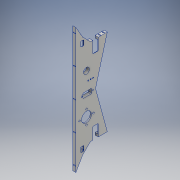
# Autodesk Inventor part: 옆판_오른쪽
Saved by Autodesk Inventor 2017 (Build 210142000, 142)
## iProperties
Part Number: 옆판_오른쪽
Material: 알루미늄 6061
Document SubType Name: Modeling
Designer: minom
Density: 2.7 g/cm^3
Appearance: 알루미늄 - 평지
Mass: 106.182 g
Surface Area: 461.014 cm^2
Volume: 39.3265 cm^3
Author: minom
Autodesk Inventor part; units mm, degrees
(part 1 of 2)
ref_plane "YZ Plane" through (0, 0, 0) normal (1, 0, 0) x (0, 1, 0)
ref_plane "XZ Plane" through (0, 0, 0) normal (0, 1, 0) x (-1, 0, 0)
ref_plane "XY Plane" through (0, 0, 0) normal (0, 0, 1) x (1, 0, 0)
sketch "스케치1" plane through (0, 0, 0) normal (1, 0, 0) x (0, 1, 0)
  line L0 (0, 0) -> (0, -320)
  line L1 (0, 0) -> (0, -50)
  line L2 (0, -50) -> (80, -50)
  line L3 (0, -320) -> (0, -270)
  line L4 (0, -270) -> (80, -270)
  line L5 (0, 0) -> (0, -30)
  line L6 (0, -30) -> (0, -50)
  line L7 (0, -320) -> (0, -290)
  line L8 (0, -290) -> (0, -270)
  line L9 (0, -290) -> (60, -290)
  line L10 (0, 0) -> (17.3205, -30)
  line L11 (0, 0) -> (34.641, 0) construction
  line L12 (17.3205, -30) -> (37.3205, -50)
  line L13 (17.3205, -30) -> (45.6048, -30) construction
  line L14 (0, -320) -> (17.3205, -290)
  line L15 (0, -320) -> (34.641, -320) construction
  line L16 (17.3205, -290) -> (37.3205, -270)
  line L17 (17.3205, -290) -> (45.6048, -290) construction
  line L18 (0, -30) -> (60, -30)
  line L19 (80, -270) -> (80, -50)
  line L20 (50, -50) -> (50, -270)
  line L21 (50, -160) -> (0, -160)
  dimension "d0" = 320
  dimension "d1" = 50
  dimension "d2" = 80
  dimension "d3" = 50
  dimension "d4" = 80
  dimension "d5" = 30
  dimension "d6" = 30
  dimension "d7" = 60
  dimension "d8" = 60
  dimension "d9" = 45
  dimension "d10" = 60
  dimension "d11" = 45
  dimension "d182" = 50
  constraints: 44 end point, 9 point on line, 6 horizontal, 4 equal length, 3 perpendicular, 2 collinear, 2 midpoint, 1 vertical
  measures "d0" distance of L0.start L0.end
  measures "d1" distance of L0.start L1.end
  measures "d2" distance of L1.end L2.end
  measures "d3" distance of L0.end L3.end
  measures "d4" distance of L3.end L4.end
  measures "d5" distance of L0.start L5.end
  measures "d6" distance of L0.end L7.end
  measures "d7" distance of L7.end L9.end
  measures "d8" angle of L10 L11
  measures "d9" angle of L12 L13
  measures "d10" angle of L15 L14
  measures "d11" angle of L17 L16
  measures "d182" distance between parallel lines of L20 L0
extrude "돌출1" add sketch "스케치1" along normal blind 8
sketch "스케치5" plane through (0, 0, 0) normal (-1, 0, 0) x (0, 0, 1)
  line L0 (-270, 80) -> (-50, 80) projected
  line L1 (-270, 80) -> (-211, 80)
  line L2 (-211, 80) -> (-211, 27)
  circle A0 centre (-211, 27) radius 21.25
  line L3 (0, 0) -> (-320, 0) projected
  dimension "d39" = 59
  dimension "d41" = 42.5
  dimension "d184" = 27
  constraints: 4 end point, 1 centre point, 1 coincident, 1 perpendicular, 1 point on line
  measures "d39" distance of L0.start L1.end
  measures "d41" diameter of A0
  measures "d184" distance from line of L3 L2.end
extrude "돌출4" cut sketch "스케치5" against normal blind 5
sketch "스케치6" plane through (5, 27, -211) normal (-1, 0, 0) x (0, 0, 1)
  circle A0 centre (0, 0) radius 21.25 projected
  line L0 (-109, -27) -> (-79, -9.6795) projected
  line L1 (211, -27) -> (-109, -27) projected
  line L2 (181, -9.6795) -> (211, -27) projected
  line L3 (161, 10.3205) -> (181, -9.6795) projected
  line L4 (161, 53) -> (161, 10.3205) projected
  line L5 (-59, 53) -> (161, 53) projected
  line L6 (-59, 10.3205) -> (-59, 53) projected
  line L7 (-79, -9.6795) -> (-59, 10.3205) projected
  line L8 (0, 0) -> (0, 17.6)
  line L9 (0, 17.6) -> (0, -17.6)
  line L10 (0, 0) -> (17.6, 0)
  line L11 (17.6, 0) -> (-17.6, 0)
  circle A1 centre (0, 17.6) radius 2.1
  circle A2 centre (17.6, 0) radius 2.1
  circle A3 centre (0, -17.6) radius 2.1
  circle A4 centre (-17.6, 0) radius 2.1
  circle A5 centre (0, 0) radius 12.6
  dimension "d44" = 17.6
  dimension "d45" = 35.2
  dimension "d46" = 17.6
  dimension "d47" = 35.2
  dimension "d48" = 4.2
  dimension "d49" = 4.2
  dimension "d50" = 4.2
  dimension "d51" = 4.2
  dimension "d52" = 25.2
  constraints: 8 end point, 5 centre point, 5 coincident, 2 point on line, 1 horizontal, 1 vertical
  measures "d44" distance of L8.start L8.end
  measures "d45" distance of L8.end L9.end
  measures "d46" distance of L8.start L10.end
  measures "d47" distance of L10.end L11.end
  measures "d48" diameter of A1
  measures "d49" diameter of A2
  measures "d50" diameter of A3
  measures "d51" diameter of A4
  measures "d52" diameter of A5
extrude "돌출5" cut sketch "스케치6" against normal blind 3 contours L11 A5 L8 | L10 A5 L9 | L8 A5 L10 | L9 A5 L11 | A1 | A2 | A3 | A4
sketch "스케치7" plane through (8, 0, 0) normal (1, 0, 0) x (0, 0, -1)
  line L0 (320, 0) -> (290, 17.3205) projected
  line L1 (290, 17.3205) -> (270, 37.3205) projected
  line L2 (270, 37.3205) -> (270, 80) projected
  line L3 (270, 80) -> (50, 80) projected
  line L4 (50, 80) -> (50, 37.3205) projected
  line L5 (50, 37.3205) -> (30, 17.3205) projected
  line L6 (30, 17.3205) -> (0, 0) projected
  line L7 (0, 0) -> (320, 0) projected
  line L8 (270, 37.3205) -> (270, 20.3205)
  line L9 (272, 20.3205) -> (281, 20.3205)
  line L10 (283, 18.3205) -> (283, 14.3205)
  line L11 (281, 12.3205) -> (272, 12.3205)
  line L12 (270, 14.3205) -> (270, 18.3205)
  line L13 (50, 37.3205) -> (50, 20.3205)
  line L14 (48, 20.3205) -> (39, 20.3205)
  line L15 (37, 18.3205) -> (37, 14.3205)
  line L16 (39, 12.3205) -> (48, 12.3205)
  line L17 (50, 14.3205) -> (50, 18.3205)
  arc A0 (39, 20.3205) -> (37, 18.3205) centre (39, 18.3205) ccw
  arc A1 (50, 18.3205) -> (48, 20.3205) centre (48, 18.3205) ccw
  arc A2 (48, 12.3205) -> (50, 14.3205) centre (48, 14.3205) ccw
  arc A3 (37, 14.3205) -> (39, 12.3205) centre (39, 14.3205) ccw
  arc A4 (272, 20.3205) -> (270, 18.3205) centre (272, 18.3205) ccw
  arc A5 (283, 18.3205) -> (281, 20.3205) centre (281, 18.3205) ccw
  arc A6 (281, 12.3205) -> (283, 14.3205) centre (281, 14.3205) ccw
  arc A7 (270, 14.3205) -> (272, 12.3205) centre (272, 14.3205) ccw
  point P0 (50, 12.3205)
  point P1 (37, 12.3205)
  point P2 (37, 20.3205)
  point P3 (270, 37.3205)
  point P4 (270, 12.3205)
  point P5 (283, 12.3205)
  point P6 (283, 20.3205)
  dimension "d55" = 17
  dimension "d56" = 8
  dimension "d57" = 13
  dimension "d61" = 17
  dimension "d62" = 13
  dimension "d63" = 8
  dimension "d142" = 2
  constraints: 20 end point, 18 point on line, 16 point on circle, 16 tangent, 8 centre point, 7 equal radius, 4 parallel, 2 horizontal, 2 perpendicular, 2 vertical
  measures "d55" distance of L8.end L1.end
  measures "d56" distance of point (283, 12.321) point (283, 20.321)
  measures "d57" distance of point (270, 12.321) point (283, 12.321)
  measures "d61" distance of L13.end L4.end
  measures "d62" distance of point (50, 12.321) point (37, 12.321)
  measures "d63" distance of point (37, 12.321) point (37, 20.321)
  measures "d142" radius of A0
extrude "돌출7" cut sketch "스케치7" against normal blind 10 contours L9 A5 L10 A6 L11 A7 L12 A4 | A1 L17 A2 L16 A3 L15 A0 L14
sketch "스케치9" plane through (0, 0, 0) normal (-1, 0, 0) x (0, 0, 1)
  line L0 (-270, 18.3205) -> (-270, 14.3205) projected
  line L1 (-272, 12.3205) -> (-281, 12.3205) projected
  line L2 (-283, 14.3205) -> (-283, 18.3205) projected
  line L3 (-281, 20.3205) -> (-272, 20.3205) projected
  line L4 (-37, 18.3205) -> (-37, 14.3205) projected
  line L5 (-39, 12.3205) -> (-48, 12.3205) projected
  line L6 (-50, 14.3205) -> (-50, 18.3205) projected
  line L7 (-48, 20.3205) -> (-39, 20.3205) projected
  circle A0 centre (-211, 27) radius 21.25 projected
  line L8 (-320, 0) -> (-290, 17.3205) projected
  line L9 (0, 0) -> (-320, 0) projected
  line L10 (-30, 17.3205) -> (0, 0) projected
  line L11 (-50, 37.3205) -> (-30, 17.3205) projected
  line L12 (-50, 80) -> (-50, 37.3205) projected
  line L13 (-270, 80) -> (-50, 80) projected
  line L14 (-270, 37.3205) -> (-270, 80) projected
  line L15 (-290, 17.3205) -> (-270, 37.3205) projected
  circle A1 centre (-109, 27) radius 7.55
  arc A2 (-270, 18.3205) -> (-272, 20.3205) centre (-272, 18.3205) ccw projected
  arc A3 (-272, 12.3205) -> (-270, 14.3205) centre (-272, 14.3205) ccw projected
  arc A4 (-283, 14.3205) -> (-281, 12.3205) centre (-281, 14.3205) ccw projected
  arc A5 (-281, 20.3205) -> (-283, 18.3205) centre (-281, 18.3205) ccw projected
  arc A6 (-37, 18.3205) -> (-39, 20.3205) centre (-39, 18.3205) ccw projected
  arc A7 (-39, 12.3205) -> (-37, 14.3205) centre (-39, 14.3205) ccw projected
  arc A8 (-50, 14.3205) -> (-48, 12.3205) centre (-48, 14.3205) ccw projected
  arc A9 (-48, 20.3205) -> (-50, 18.3205) centre (-48, 18.3205) ccw projected
  dimension "d67" = 15.1
  dimension "d68" = 102
  dimension "d185" = 27
  constraints: 1 centre point
  measures "d67" diameter of A1
  measures "d68" distance of A1.centre A0.centre
  measures "d185" distance from line of L9 A1.centre
extrude "돌출8" cut sketch "스케치9" against normal blind 10 contours A1
sketch "스케치10" plane through (8, 0, 0) normal (1, 0, 0) x (0, 0, -1)
  circle A0 centre (109, 27) radius 7.55 projected
  line L0 (270, 18.3205) -> (270, 14.3205) projected
  line L1 (272, 12.3205) -> (281, 12.3205) projected
  line L2 (283, 14.3205) -> (283, 18.3205) projected
  line L3 (281, 20.3205) -> (272, 20.3205) projected
  line L4 (37, 18.3205) -> (37, 14.3205) projected
  line L5 (39, 12.3205) -> (48, 12.3205) projected
  line L6 (50, 14.3205) -> (50, 18.3205) projected
  line L7 (48, 20.3205) -> (39, 20.3205) projected
  circle A1 centre (211, 27) radius 21.25 projected
  line L8 (320, 0) -> (290, 17.3205) projected
  line L9 (0, 0) -> (320, 0) projected
  line L10 (30, 17.3205) -> (0, 0) projected
  line L11 (50, 37.3205) -> (30, 17.3205) projected
  line L12 (50, 80) -> (50, 37.3205) projected
  line L13 (270, 80) -> (50, 80) projected
  line L14 (270, 37.3205) -> (270, 80) projected
  line L15 (290, 17.3205) -> (270, 37.3205) projected
  circle A2 centre (109, 27) radius 7.55 projected
  line L16 (272, 20.3205) -> (281, 20.3205) projected
  line L17 (283, 18.3205) -> (283, 14.3205) projected
  line L18 (281, 12.3205) -> (272, 12.3205) projected
  line L19 (270, 14.3205) -> (270, 18.3205) projected
  line L20 (39, 20.3205) -> (48, 20.3205) projected
  line L21 (50, 18.3205) -> (50, 14.3205) projected
  line L22 (48, 12.3205) -> (39, 12.3205) projected
  line L23 (37, 14.3205) -> (37, 18.3205) projected
  circle A3 centre (228.6, 27) radius 2.1 projected
  circle A4 centre (193.4, 27) radius 2.1 projected
  circle A5 centre (211, 44.6) radius 2.1 projected
  circle A6 centre (211, 9.4) radius 2.1 projected
  circle A7 centre (211, 27) radius 12.6 projected
  line L24 (320, 0) -> (290, 17.3205) projected
  line L25 (290, 17.3205) -> (270, 37.3205) projected
  line L26 (270, 37.3205) -> (270, 80) projected
  line L27 (270, 80) -> (50, 80) projected
  line L28 (50, 80) -> (50, 37.3205) projected
  line L29 (50, 37.3205) -> (30, 17.3205) projected
  line L30 (30, 17.3205) -> (0, 0) projected
  line L31 (0, 0) -> (320, 0) projected
  line L32 (156, 40) -> (164, 40)
  line L33 (166, 38) -> (166, 20)
  line L34 (164, 18) -> (156, 18)
  line L35 (154, 20) -> (154, 38)
  arc A8 (166, 38) -> (164, 40) centre (164, 38) ccw
  arc A9 (164, 18) -> (166, 20) centre (164, 20) ccw
  arc A10 (154, 20) -> (156, 18) centre (156, 20) ccw
  arc A11 (156, 40) -> (154, 38) centre (156, 38) ccw
  arc A12 (272, 20.3205) -> (270, 18.3205) centre (272, 18.3205) ccw projected
  arc A13 (283, 18.3205) -> (281, 20.3205) centre (281, 18.3205) ccw projected
  arc A14 (281, 12.3205) -> (283, 14.3205) centre (281, 14.3205) ccw projected
  arc A15 (270, 14.3205) -> (272, 12.3205) centre (272, 14.3205) ccw projected
  arc A16 (39, 20.3205) -> (37, 18.3205) centre (39, 18.3205) ccw projected
  arc A17 (50, 18.3205) -> (48, 20.3205) centre (48, 18.3205) ccw projected
  arc A18 (48, 12.3205) -> (50, 14.3205) centre (48, 14.3205) ccw projected
  arc A19 (37, 14.3205) -> (39, 12.3205) centre (39, 14.3205) ccw projected
  arc A20 (272, 20.3205) -> (270, 18.3205) centre (272, 18.3205) ccw projected
  arc A21 (270, 14.3205) -> (272, 12.3205) centre (272, 14.3205) ccw projected
  arc A22 (281, 12.3205) -> (283, 14.3205) centre (281, 14.3205) ccw projected
  arc A23 (283, 18.3205) -> (281, 20.3205) centre (281, 18.3205) ccw projected
  arc A24 (39, 20.3205) -> (37, 18.3205) centre (39, 18.3205) ccw projected
  arc A25 (37, 14.3205) -> (39, 12.3205) centre (39, 14.3205) ccw projected
  arc A26 (48, 12.3205) -> (50, 14.3205) centre (48, 14.3205) ccw projected
  arc A27 (50, 18.3205) -> (48, 20.3205) centre (48, 18.3205) ccw projected
  point P0 (166, 18)
  point P1 (166, 40)
  point P2 (154, 18)
  dimension "d71" = 12
  dimension "d72" = 22
  dimension "d73" = 104
  dimension "d74" = 40
  dimension "d75" = 2
  constraints: 8 end point, 8 point on circle, 8 tangent, 6 point on line, 4 centre point, 3 equal radius, 2 parallel, 1 horizontal, 1 perpendicular
  measures "d71" distance of point (166, 18) point (154, 18)
  measures "d72" distance of point (166, 40) point (166, 18)
  measures "d73" distance between parallel lines of L35 L12
  measures "d74" distance between parallel lines of L13 L32
  measures "d75" radius of A8
extrude "돌출9" cut sketch "스케치10" against normal blind 10 contours L32 A8 L33 A9 L34 A10 L35 A11
sketch "스케치11" plane through (0, 0, -320) normal (0, -1, 0) x (1, 0, 0)
  line L0 (0, 320) -> (0, 0) projected
  line L1 (0, 0) -> (8, 0) projected
  line L2 (8, 320) -> (8, 0) projected
  line L3 (0, 320) -> (8, 320) projected
  line L4 (0, 320) -> (8, 320) projected
  line L5 (4, 320) -> (4, 306)
  line L6 (4, 306) -> (4, 233)
  line L7 (4, 233) -> (4, 160)
  line L8 (4, 160) -> (4, 87)
  line L9 (4, 87) -> (4, 14)
  line L10 (4, 14) -> (4, 0)
  circle A0 centre (4, 306) radius 1.25
  circle A1 centre (4, 233) radius 1.25
  circle A2 centre (4, 160) radius 1.25
  circle A3 centre (4, 87) radius 1.25
  circle A4 centre (4, 14) radius 1.25
  dimension "d78" = 14
  dimension "d79" = 73
  dimension "d80" = 73
  dimension "d81" = 73
  dimension "d82" = 73
  dimension "d83" = 2.5
  dimension "d84" = 2.5
  dimension "d85" = 2.5
  dimension "d86" = 2.5
  dimension "d87" = 2.5
  constraints: 12 end point, 5 centre point, 5 coincident, 4 point on line, 2 midpoint, 1 vertical
  measures "d78" distance of L5.start L5.end
  measures "d79" distance of L5.end L6.end
  measures "d80" distance of L6.end L7.end
  measures "d81" distance of L7.end L8.end
  measures "d82" distance of L8.end L9.end
  measures "d83" diameter of A0
  measures "d84" diameter of A1
  measures "d85" diameter of A2
  measures "d86" diameter of A3
  measures "d87" diameter of A4
sketch "스케치12" plane through (0, 0, 0) normal (-1, 0, 0) x (0, 0, 1)
  arc A0 (-164, 40) -> (-166, 38) centre (-164, 38) ccw projected
  line L0 (-164, 40) -> (-156, 40) projected
  arc A1 (-154, 38) -> (-156, 40) centre (-156, 38) ccw projected
  line L1 (-154, 38) -> (-154, 20) projected
  arc A2 (-156, 18) -> (-154, 20) centre (-156, 20) ccw projected
  line L2 (-156, 18) -> (-164, 18) projected
  arc A3 (-166, 20) -> (-164, 18) centre (-164, 20) ccw projected
  line L3 (-166, 20) -> (-166, 38) projected
  circle A4 centre (-109, 27) radius 7.55 projected
  line L4 (-270, 18.3205) -> (-270, 14.3205) projected
  line L5 (-272, 12.3205) -> (-281, 12.3205) projected
  line L6 (-283, 14.3205) -> (-283, 18.3205) projected
  line L7 (-281, 20.3205) -> (-272, 20.3205) projected
  line L8 (-37, 18.3205) -> (-37, 14.3205) projected
  line L9 (-39, 12.3205) -> (-48, 12.3205) projected
  line L10 (-50, 14.3205) -> (-50, 18.3205) projected
  line L11 (-48, 20.3205) -> (-39, 20.3205) projected
  circle A5 centre (-211, 27) radius 21.25 projected
  line L12 (-320, 0) -> (-290, 17.3205) projected
  line L13 (0, 0) -> (-320, 0) projected
  line L14 (-30, 17.3205) -> (0, 0) projected
  line L15 (-50, 37.3205) -> (-30, 17.3205) projected
  line L16 (-50, 80) -> (-50, 37.3205) projected
  line L17 (-270, 80) -> (-50, 80) projected
  line L18 (-270, 37.3205) -> (-270, 80) projected
  line L19 (-290, 17.3205) -> (-270, 37.3205) projected
  circle A6 centre (-160, 43.5) radius 1.5
  circle A7 centre (-160, 14.5) radius 1.5
  arc A8 (-270, 18.3205) -> (-272, 20.3205) centre (-272, 18.3205) ccw projected
  arc A9 (-272, 12.3205) -> (-270, 14.3205) centre (-272, 14.3205) ccw projected
  arc A10 (-283, 14.3205) -> (-281, 12.3205) centre (-281, 14.3205) ccw projected
  arc A11 (-281, 20.3205) -> (-283, 18.3205) centre (-281, 18.3205) ccw projected
  arc A12 (-37, 18.3205) -> (-39, 20.3205) centre (-39, 18.3205) ccw projected
  arc A13 (-39, 12.3205) -> (-37, 14.3205) centre (-39, 14.3205) ccw projected
  arc A14 (-50, 14.3205) -> (-48, 12.3205) centre (-48, 14.3205) ccw projected
  arc A15 (-48, 20.3205) -> (-50, 18.3205) centre (-48, 18.3205) ccw projected
  dimension "d90" = 3
  dimension "d91" = 3
  dimension "d92" = 3.5
  dimension "d93" = 3.5
  dimension "d94" = 6
  dimension "d95" = 6
  constraints: 2 centre point
  measures "d90" diameter of A6
  measures "d91" diameter of A7
  measures "d92" distance from line of L2 A7.centre
  measures "d93" distance from line of L0 A6.centre
  measures "d94" distance from line of L3 A6.centre
  measures "d95" distance from line of L1 A7.centre
extrude "돌출11" cut sketch "스케치12" against normal blind 10 contours A6 | A7
sketch "스케치13" plane through (8, 0, 0) normal (1, 0, 0) x (0, 0, -1)
  circle A0 centre (160, 43.5) radius 1.5 projected
  circle A1 centre (160, 14.5) radius 1.5 projected
  arc A2 (166, 38) -> (164, 40) centre (164, 38) ccw projected
  line L0 (166, 38) -> (166, 20) projected
  arc A3 (164, 18) -> (166, 20) centre (164, 20) ccw projected
  line L1 (164, 18) -> (156, 18) projected
  arc A4 (154, 20) -> (156, 18) centre (156, 20) ccw projected
  line L2 (154, 20) -> (154, 38) projected
  arc A5 (156, 40) -> (154, 38) centre (156, 38) ccw projected
  line L3 (156, 40) -> (164, 40) projected
  circle A6 centre (109, 27) radius 7.55 projected
  line L4 (272, 20.3205) -> (281, 20.3205) projected
  line L5 (283, 18.3205) -> (283, 14.3205) projected
  line L6 (281, 12.3205) -> (272, 12.3205) projected
  line L7 (270, 14.3205) -> (270, 18.3205) projected
  line L8 (39, 20.3205) -> (48, 20.3205) projected
  line L9 (50, 18.3205) -> (50, 14.3205) projected
  line L10 (48, 12.3205) -> (39, 12.3205) projected
  line L11 (37, 14.3205) -> (37, 18.3205) projected
  circle A7 centre (228.6, 27) radius 2.1 projected
  circle A8 centre (193.4, 27) radius 2.1 projected
  circle A9 centre (211, 44.6) radius 2.1 projected
  circle A10 centre (211, 9.4) radius 2.1 projected
  circle A11 centre (211, 27) radius 12.6 projected
  line L12 (320, 0) -> (290, 17.3205) projected
  line L13 (290, 17.3205) -> (270, 37.3205) projected
  line L14 (270, 37.3205) -> (270, 80) projected
  line L15 (270, 80) -> (50, 80) projected
  line L16 (50, 80) -> (50, 37.3205) projected
  line L17 (50, 37.3205) -> (30, 17.3205) projected
  line L18 (30, 17.3205) -> (0, 0) projected
  line L19 (0, 0) -> (320, 0) projected
  line L20 (50, 80) -> (50, 37.3205) projected
  line L21 (50, 57) -> (78, 57)
  line L22 (80, 55) -> (80, 45)
  line L23 (78, 43) -> (50, 43)
  line L24 (50, 43) -> (50, 57)
  line L25 (270, 37.3205) -> (270, 80) projected
  line L26 (270, 57) -> (242, 57)
  line L27 (240, 55) -> (240, 45)
  line L28 (242, 43) -> (270, 43)
  line L29 (270, 43) -> (270, 57)
  arc A12 (272, 20.3205) -> (270, 18.3205) centre (272, 18.3205) ccw projected
  arc A13 (283, 18.3205) -> (281, 20.3205) centre (281, 18.3205) ccw projected
  arc A14 (281, 12.3205) -> (283, 14.3205) centre (281, 14.3205) ccw projected
  arc A15 (270, 14.3205) -> (272, 12.3205) centre (272, 14.3205) ccw projected
  arc A16 (39, 20.3205) -> (37, 18.3205) centre (39, 18.3205) ccw projected
  arc A17 (50, 18.3205) -> (48, 20.3205) centre (48, 18.3205) ccw projected
  arc A18 (48, 12.3205) -> (50, 14.3205) centre (48, 14.3205) ccw projected
  arc A19 (37, 14.3205) -> (39, 12.3205) centre (39, 14.3205) ccw projected
  arc A20 (242, 57) -> (240, 55) centre (242, 55) ccw
  arc A21 (240, 45) -> (242, 43) centre (242, 45) ccw
  arc A22 (80, 55) -> (78, 57) centre (78, 55) ccw
  arc A23 (78, 43) -> (80, 45) centre (78, 45) ccw
  point P0 (80, 43)
  point P1 (80, 57)
  point P2 (240, 43)
  point P3 (240, 57)
  dimension "d98" = 30
  dimension "d99" = 14
  dimension "d100" = 23
  dimension "d101" = 30
  dimension "d102" = 14
  dimension "d103" = 23
  dimension "d181" = 2
  constraints: 16 end point, 10 point on line, 8 point on circle, 8 tangent, 4 centre point, 4 parallel, 3 equal radius, 2 horizontal, 2 perpendicular
  measures "d98" distance of point (80, 43) L23.end
  measures "d99" distance of point (80, 57) point (80, 43)
  measures "d100" distance between parallel lines of L21 L15
  measures "d101" distance of L28.end point (240, 43)
  measures "d102" distance of point (240, 43) point (240, 57)
  measures "d103" distance between parallel lines of L26 L15
  measures "d181" radius of A20
extrude "돌출12" cut sketch "스케치13" against normal blind 10 contours L28 A21 L27 A20 L26 L14 | L16 L21 A22 L22 A23 L23
sketch "스케치15" plane through (0, 17.3205, -30) normal (0, 0.7071068, 0.7071068) x (1, 0, 0)
  circle A0 centre (44, 8) radius 1.6 projected
  circle A1 centre (4, 18) radius 1.6 projected
  circle A2 centre (-215.8, 18) radius 1.6 projected
  circle A3 centre (-255.8, 18) radius 1.6 projected
  circle A4 centre (-255.8, 8) radius 1.6 projected
  circle A5 centre (-215.8, 8) radius 1.6 projected
  circle A6 centre (4, 8) radius 1.6 projected
  circle A7 centre (44, 18) radius 1.6 projected
  line L0 (-260.9, 27) -> (49.1, 27) projected
  line L1 (-260.9, 1) -> (-260.9, 27) projected
  line L2 (49.1, 1) -> (-97.9, 1) projected
  line L3 (-113.9, 1) -> (-260.9, 1) projected
  line L4 (49.1, 27) -> (49.1, 1) projected
  circle A8 centre (4, 18) radius 1.25
  circle A9 centre (4, 8) radius 1.25
  line L5 (-113.9, 1) -> (-113.9, 8) projected
  arc A10 (-111.9, 10) -> (-113.9, 8) centre (-111.9, 8) ccw projected
  line L6 (-111.9, 10) -> (-99.9, 10) projected
  arc A11 (-97.9, 8) -> (-99.9, 10) centre (-99.9, 8) ccw projected
  line L7 (-97.9, 8) -> (-97.9, 1) projected
  circle A12 centre (-148.8, 18) radius 1.6 projected
  circle A13 centre (-63, 8) radius 1.6 projected
  circle A14 centre (-63, 18) radius 1.6 projected
  circle A15 centre (-148.8, 8) radius 1.6 projected
  point P0 (0, -33.4607)
  dimension "d110" = 2.5
  dimension "d111" = 2.5
  constraints: 2 centre point, 2 coincident
  measures "d110" diameter of A8
  measures "d111" diameter of A9
sketch "스케치18" plane through (8, 37.3205, -270) normal (0, 0.7071068, -0.7071068) x (-1, 0, 0)
  circle A0 centre (263.8, -20.2641) radius 1.6 projected
  circle A1 centre (223.8, -10.2641) radius 1.6 projected
  circle A2 centre (4, -10.2641) radius 1.6 projected
  circle A3 centre (-36, -10.2641) radius 1.6 projected
  circle A4 centre (-36, -20.2641) radius 1.6 projected
  circle A5 centre (4, -20.2641) radius 1.6 projected
  circle A6 centre (223.8, -20.2641) radius 1.6 projected
  circle A7 centre (263.8, -10.2641) radius 1.6 projected
  line L0 (-41.1, -1.2641) -> (268.9, -1.2641) projected
  line L1 (-41.1, -27.2641) -> (-41.1, -1.2641) projected
  line L2 (268.9, -27.2641) -> (121.9, -27.2641) projected
  line L3 (105.9, -27.2641) -> (-41.1, -27.2641) projected
  line L4 (268.9, -1.2641) -> (268.9, -27.2641) projected
  circle A8 centre (4, -10.2641) radius 1.25
  circle A9 centre (4, -20.2641) radius 1.25
  line L5 (105.9, -27.2641) -> (105.9, -20.2641) projected
  arc A10 (107.9, -18.2641) -> (105.9, -20.2641) centre (107.9, -20.2641) ccw projected
  line L6 (107.9, -18.2641) -> (119.9, -18.2641) projected
  arc A11 (121.9, -20.2641) -> (119.9, -18.2641) centre (119.9, -20.2641) ccw projected
  line L7 (121.9, -20.2641) -> (121.9, -27.2641) projected
  circle A12 centre (71, -10.2641) radius 1.6 projected
  circle A13 centre (156.8, -20.2641) radius 1.6 projected
  circle A14 centre (156.8, -10.2641) radius 1.6 projected
  circle A15 centre (71, -20.2641) radius 1.6 projected
  point P0 (8, 164.5292)
  dimension "d122" = 2.5
  dimension "d123" = 2.5
  constraints: 2 centre point, 2 coincident
  measures "d122" diameter of A8
  measures "d123" diameter of A9
sketch "스케치22" plane through (8, 0, 0) normal (1, 0, 0) x (0, 0, -1)
  line L0 (50, 80) -> (50, 37.3205) projected
  line L1 (50, 50) -> (270, 50)
  line L2 (270, 37.3205) -> (270, 43) projected
  circle A0 centre (211, 27) radius 12.6 projected
  circle A1 centre (211, 9.4) radius 2.1 projected
  circle A2 centre (211, 44.6) radius 2.1 projected
  circle A3 centre (193.4, 27) radius 2.1 projected
  circle A4 centre (228.6, 27) radius 2.1 projected
  arc A5 (39, 20.3205) -> (37, 18.3205) centre (39, 18.3205) ccw projected
  line L3 (39, 20.3205) -> (48, 20.3205) projected
  arc A6 (50, 18.3205) -> (48, 20.3205) centre (48, 18.3205) ccw projected
  line L4 (50, 18.3205) -> (50, 14.3205) projected
  arc A7 (48, 12.3205) -> (50, 14.3205) centre (48, 14.3205) ccw projected
  line L5 (48, 12.3205) -> (39, 12.3205) projected
  arc A8 (37, 14.3205) -> (39, 12.3205) centre (39, 14.3205) ccw projected
  line L6 (37, 14.3205) -> (37, 18.3205) projected
  arc A9 (272, 20.3205) -> (270, 18.3205) centre (272, 18.3205) ccw projected
  line L7 (272, 20.3205) -> (281, 20.3205) projected
  arc A10 (283, 18.3205) -> (281, 20.3205) centre (281, 18.3205) ccw projected
  line L8 (283, 18.3205) -> (283, 14.3205) projected
  arc A11 (281, 12.3205) -> (283, 14.3205) centre (281, 14.3205) ccw projected
  line L9 (281, 12.3205) -> (272, 12.3205) projected
  arc A12 (270, 14.3205) -> (272, 12.3205) centre (272, 14.3205) ccw projected
  line L10 (270, 14.3205) -> (270, 18.3205) projected
  circle A13 centre (109, 27) radius 7.55 projected
  arc A14 (166, 38) -> (164, 40) centre (164, 38) ccw projected
  line L11 (166, 38) -> (166, 20) projected
  arc A15 (164, 18) -> (166, 20) centre (164, 20) ccw projected
  line L12 (164, 18) -> (156, 18) projected
  arc A16 (154, 20) -> (156, 18) centre (156, 20) ccw projected
  line L13 (154, 20) -> (154, 38) projected
  arc A17 (156, 40) -> (154, 38) centre (156, 38) ccw projected
  line L14 (156, 40) -> (164, 40) projected
  circle A18 centre (160, 14.5) radius 1.5 projected
  circle A19 centre (160, 43.5) radius 1.5 projected
  line L15 (30, 17.3205) -> (0, 0) projected
  line L16 (0, 0) -> (320, 0) projected
  line L17 (320, 0) -> (290, 17.3205) projected
  line L18 (290, 17.3205) -> (270, 37.3205) projected
  line L19 (270, 37.3205) -> (270, 43) projected
  line L20 (270, 43) -> (242, 43) projected
  arc A20 (240, 45) -> (242, 43) centre (242, 45) ccw projected
  line L21 (240, 45) -> (240, 55) projected
  arc A21 (242, 57) -> (240, 55) centre (242, 55) ccw projected
  line L22 (242, 57) -> (270, 57) projected
  line L23 (270, 80) -> (50, 80) projected
  line L24 (50, 80) -> (50, 57) projected
  line L25 (50, 57) -> (78, 57) projected
  arc A22 (80, 55) -> (78, 57) centre (78, 55) ccw projected
  line L26 (80, 55) -> (80, 45) projected
  arc A23 (78, 43) -> (80, 45) centre (78, 45) ccw projected
  line L27 (78, 43) -> (50, 43) projected
  line L28 (50, 37.3205) -> (30, 17.3205) projected
  line L29 (50, 80) -> (50, 65.6614) projected
  line L30 (50, 80) -> (160, 50)
  line L31 (270, 80) -> (248.6614, 80) projected
  line L32 (160, 50) -> (270, 80)
  line L33 (270, 57) -> (270, 80) projected
  line L34 (50, 43) -> (50, 37.3205) projected
  point P0 (50, 42.3386)
  point P1 (270, 42.3386)
  point P2 (248.6614, 70)
  constraints: 6 end point, 2 point on line, 1 horizontal, 1 midpoint
extrude "돌출22" cut sketch "스케치22" against normal blind 8 contours L23 L32 L30
sketch "스케치24" plane through (0, 0, 0) normal (-1, 0, 0) x (0, 0, 1)
  line L0 (-160, 50) -> (-270, 80) projected
  line L1 (-270, 57) -> (-270, 80) projected
  line L2 (-270, 57) -> (-242, 57) projected
  arc A0 (-240, 55) -> (-242, 57) centre (-242, 55) ccw projected
  line L3 (-240, 55) -> (-240, 45) projected
  arc A1 (-242, 43) -> (-240, 45) centre (-242, 45) ccw projected
  line L4 (-242, 43) -> (-270, 43) projected
  line L5 (-270, 37.3205) -> (-270, 43) projected
  line L6 (-290, 17.3205) -> (-270, 37.3205) projected
  line L7 (-320, 0) -> (-290, 17.3205) projected
  line L8 (0, 0) -> (-320, 0) projected
  line L9 (-30, 17.3205) -> (0, 0) projected
  line L10 (-50, 37.3205) -> (-30, 17.3205) projected
  line L11 (-50, 43) -> (-50, 37.3205) projected
  line L12 (-50, 43) -> (-78, 43) projected
  arc A2 (-80, 45) -> (-78, 43) centre (-78, 45) ccw projected
  line L13 (-80, 45) -> (-80, 55) projected
  arc A3 (-78, 57) -> (-80, 55) centre (-78, 55) ccw projected
  line L14 (-78, 57) -> (-50, 57) projected
  line L15 (-50, 80) -> (-50, 57) projected
  line L16 (-50, 80) -> (-160, 50) projected
  circle A4 centre (-211, 27) radius 21.25 projected
  arc A5 (-37, 18.3205) -> (-39, 20.3205) centre (-39, 18.3205) ccw projected
  line L17 (-37, 18.3205) -> (-37, 14.3205) projected
  arc A6 (-39, 12.3205) -> (-37, 14.3205) centre (-39, 14.3205) ccw projected
  line L18 (-39, 12.3205) -> (-48, 12.3205) projected
  arc A7 (-50, 14.3205) -> (-48, 12.3205) centre (-48, 14.3205) ccw projected
  line L19 (-50, 14.3205) -> (-50, 18.3205) projected
  arc A8 (-48, 20.3205) -> (-50, 18.3205) centre (-48, 18.3205) ccw projected
  line L20 (-48, 20.3205) -> (-39, 20.3205) projected
  arc A9 (-270, 18.3205) -> (-272, 20.3205) centre (-272, 18.3205) ccw projected
  line L21 (-270, 18.3205) -> (-270, 14.3205) projected
  arc A10 (-272, 12.3205) -> (-270, 14.3205) centre (-272, 14.3205) ccw projected
  line L22 (-272, 12.3205) -> (-281, 12.3205) projected
  arc A11 (-283, 14.3205) -> (-281, 12.3205) centre (-281, 14.3205) ccw projected
  line L23 (-283, 14.3205) -> (-283, 18.3205) projected
  arc A12 (-281, 20.3205) -> (-283, 18.3205) centre (-281, 18.3205) ccw projected
  line L24 (-281, 20.3205) -> (-272, 20.3205) projected
  circle A13 centre (-109, 27) radius 7.55 projected
  arc A14 (-164, 40) -> (-166, 38) centre (-164, 38) ccw projected
  line L25 (-164, 40) -> (-156, 40) projected
  arc A15 (-154, 38) -> (-156, 40) centre (-156, 38) ccw projected
  line L26 (-154, 38) -> (-154, 20) projected
  arc A16 (-156, 18) -> (-154, 20) centre (-156, 20) ccw projected
  line L27 (-156, 18) -> (-164, 18) projected
  arc A17 (-166, 20) -> (-164, 18) centre (-164, 20) ccw projected
  line L28 (-166, 20) -> (-166, 38) projected
  circle A18 centre (-160, 14.5) radius 1.5 projected
  circle A19 centre (-109, 27) radius 7.55 projected
  line L29 (-160, 50) -> (-50, 80) projected
  line L30 (-154, 20) -> (-154, 38) projected
  line L31 (-50, 37.3205) -> (-30, 17.3205) projected
  line L32 (-166, 20) -> (-166, 38) projected
  line L33 (-160, 50) -> (-270, 80) projected
  line L34 (-267, 76.0722) -> (-267, 57)
  line L35 (-267, 43) -> (-267, 36.0779)
  line L36 (-288.158, 14.9199) -> (-308.8038, 3)
  line L37 (-11.1962, 3) -> (-31.842, 14.9199)
  line L38 (-119.2156, 29.6353) -> (-151.073, 29.6353)
  line L39 (-53, 36.0779) -> (-53, 43)
  arc A20 (-164.4696, 15.0221) -> (-155.5304, 15.0221) centre (-160, 14.5) ccw
  line L40 (-119.4428, 25.5) -> (-151, 25.5)
  line L41 (-98.5572, 25.5) -> (-42.4221, 25.5)
  line L42 (-53, 57) -> (-53, 76.0722)
  line L43 (-113.4025, 59.5988) -> (-53, 76.0722)
  line L44 (-206.5975, 59.5988) -> (-267, 76.0722)
  line L45 (-235.2036, 28.5) -> (-274.5779, 28.5)
  line L46 (-235.2036, 25.5) -> (-277.5779, 25.5)
  line L47 (-208.1461, 51.0815) -> (-206.5975, 59.5988)
  line L48 (-205.1945, 50.5448) -> (-203.6924, 58.8065)
  line L49 (-186.7964, 28.5) -> (-168.975, 28.5)
  line L50 (-186.7964, 25.5) -> (-169, 25.5)
  line L51 (-308.8038, 3) -> (-214.4731, 3)
  line L52 (-162.2597, 47.5067) -> (-203.6924, 58.8065)
  arc A21 (-207.5269, 3) -> (-186.7964, 25.5) centre (-211, 27) ccw
  arc A22 (-186.7964, 28.5) -> (-205.1945, 50.5448) centre (-211, 27) ccw
  arc A23 (-208.1461, 51.0815) -> (-235.2036, 28.5) centre (-211, 27) ccw
  arc A24 (-235.2036, 25.5) -> (-214.4731, 3) centre (-211, 27) ccw
  line L53 (-267, 36.0779) -> (-274.5779, 28.5)
  line L54 (-277.5779, 25.5) -> (-288.158, 14.9199)
  line L55 (-157.7403, 47.5067) -> (-116.3076, 58.8065)
  line L56 (-112.3439, 37.006) -> (-116.3076, 58.8065)
  line L57 (-110.5, 16.5572) -> (-110.5, 3)
  line L58 (-107.5, 16.5572) -> (-107.5, 3)
  line L59 (-109.3923, 37.5427) -> (-113.4025, 59.5988)
  arc A25 (-107.5, 16.5572) -> (-98.5572, 25.5) centre (-109, 27) ccw
  arc A26 (-98.5572, 28.5) -> (-109.3923, 37.5427) centre (-109, 27) ccw
  arc A27 (-112.3439, 37.006) -> (-119.2156, 29.6353) centre (-109, 27) ccw
  arc A28 (-119.4428, 25.5) -> (-110.5, 16.5572) centre (-109, 27) ccw
  line L60 (-207.5269, 3) -> (-110.5, 3)
  line L61 (-107.5, 3) -> (-11.1962, 3)
  line L62 (-98.5572, 28.5) -> (-45.4221, 28.5)
  line L63 (-53, 36.0779) -> (-45.4221, 28.5)
  line L64 (-42.4221, 25.5) -> (-31.842, 14.9199)
  line L65 (-156, 18) -> (-164, 18) projected
  line L66 (-164, 40) -> (-156, 40) projected
  arc A29 (-155.5304, 15.0221) -> (-151, 20) centre (-156, 20) ccw
  arc A30 (-169, 20) -> (-164.4696, 15.0221) centre (-164, 20) ccw
  arc A31 (-151.073, 38.8515) -> (-155.4309, 42.9675) centre (-156, 38) ccw
  arc A32 (-164.5691, 42.9675) -> (-168.975, 38.4992) centre (-164, 38) ccw
  line L67 (-151.073, 38.8515) -> (-151.073, 29.6353)
  line L68 (-151, 25.5) -> (-151, 20)
  line L69 (-169, 20) -> (-169, 25.5)
  line L70 (-168.975, 28.5) -> (-168.975, 38.4992)
  circle A33 centre (-160, 43.5) radius 1.5 projected
  arc A34 (-155.4309, 42.9675) -> (-157.7403, 47.5067) centre (-160, 43.5) ccw
  arc A35 (-162.2597, 47.5067) -> (-164.5691, 42.9675) centre (-160, 43.5) ccw
  dimension "d206" = 3
  dimension "d215" = 3
  dimension "d217" = 3
  dimension "d223" = 3
  dimension "d225" = 3
  dimension "d226" = 3
  dimension "d233" = 3
  dimension "d239" = 3
  dimension "d240" = 3
  dimension "d241" = 3
  dimension "d242" = 3
  dimension "d285" = 3
  dimension "d286" = 3
  dimension "d287" = 3
  dimension "d288" = 3
  constraints: 70 end point, 30 point on circle, 15 centre point, 10 parallel, 4 point on line, 1 other
  measures "d206" distance between parallel lines of L34 L1
  measures "d215" distance between parallel lines of L11 L39
  measures "d217" radial gap between concentric circles of A18 A20
  measures "d223" distance between parallel lines of L9 L37
  measures "d225" distance between parallel lines of L15 L42
  measures "d226" distance between parallel lines of L16 L43
  measures "d233" distance between parallel lines of L33 L44
  measures "d239" radial gap between concentric circles of A16 A29
  measures "d240" radial gap between concentric circles of A17 A30
  measures "d241" radial gap between concentric circles of A15 A31
  measures "d242" radial gap between concentric circles of A14 A32
  measures "d285" distance between parallel lines of L33 L52
  measures "d286" distance between parallel lines of L55 L16
  measures "d287" distance between parallel lines of L59 L56
  measures "d288" radial gap between concentric circles of A27 A13
extrude "돌출32" cut sketch "스케치24" against normal blind 7.3 contours L34 L44 L47 A23 L45 L53 L35 L4 A1 L3 A0 L2 | L14 A3 L13 A2 L12 L39 L63 L62 A26 L59 L43 L42 | L54 L46 A24 L51 L36 | L61 L58 A25 L41 L64 L37 | L38 L67 A31 A34 L55 L56 A27 | A20 A29 L68 L40 A28 L57 L60 A21 L50 L69 A30 | L48 L52 A35 A32 L70 L49 A22
sketch "스케치25" plane through (0, 0, 0) normal (-1, 0, 0) x (0, 0, 1)
  line L0 (-158.5, 3) -> (-161.5, 3) projected
  line L1 (-158.5, 0) -> (-161.5, 0) projected
  line L2 (-85.5, 3) -> (-88.5, 3) projected
  line L3 (-85.5, 0) -> (-88.5, 0) projected
  line L4 (-12.5, 3) -> (-15.5, 3) projected
  line L5 (-12.5, 0) -> (-15.5, 0) projected
  line L6 (-231.5, 3) -> (-234.5, 3) projected
  line L7 (-231.5, 0) -> (-234.5, 0) projected
  line L8 (-304.5, 3) -> (-307.5, 3) projected
  line L9 (-304.5, 0) -> (-307.5, 0) projected
  line L10 (-308.8038, 3) -> (-307.118, 3.9733) projected
  line L11 (-307.118, 3.9733) -> (-307.118, 3.9733) projected
  line L12 (-307.118, 3.9733) -> (-308.8038, 3) projected
  line L13 (-308.8038, 3) -> (-308.6038, 3) projected
  line L14 (-308.6038, 3) -> (-308.6038, 3) projected
  line L15 (-308.6038, 3) -> (-308.8038, 3) projected
  line L16 (-310.8853, 5.2624) -> (-308.2872, 6.7624) projected
  line L17 (-298.7609, 12.2624) -> (-296.1629, 13.7624) projected
  line L18 (-297.2609, 9.6643) -> (-294.6629, 11.1643) projected
  line L19 (-298.7609, 12.2624) -> (-296.1629, 13.7624) projected
  line L20 (-283.2682, 19.8097) -> (-281.1469, 21.931) projected
  line L21 (-285.3895, 21.931) -> (-283.2682, 24.0523) projected
  line L22 (-274.5779, 28.5) -> (-274.4364, 28.5) projected
  line L23 (-274.4364, 28.5) -> (-274.4364, 28.5) projected
  line L24 (-274.4364, 28.5) -> (-274.5779, 28.5) projected
  line L25 (-274.5779, 28.5) -> (-274.5779, 28.5) projected
  line L26 (-278.3185, 29.0021) -> (-276.1971, 31.1234) projected
  line L27 (-267, 41.5) -> (-267, 44.5) projected
  line L28 (-270, 41.5) -> (-270, 44.5) projected
  line L29 (-270, 63.5) -> (-270, 66.5) projected
  line L30 (-264, 65.8599) -> (-267, 66.4054) projected
  line L31 (-267, 66.4054) -> (-267, 66.4054) projected
  line L32 (-267, 66.4054) -> (-264, 65.8599) projected
  line L33 (-264, 65.8599) -> (-264, 65.8599) projected
  line L34 (-53, 66.4054) -> (-56, 65.8599) projected
  line L35 (-56, 65.8599) -> (-56, 65.8599) projected
  line L36 (-56, 65.8599) -> (-53, 66.4054) projected
  line L37 (-53, 66.4054) -> (-53, 66.4054) projected
  line L38 (-50, 66.5) -> (-50, 63.5) projected
  line L39 (-53, 44.5) -> (-53, 41.5) projected
  line L40 (-50, 44.5) -> (-50, 41.5) projected
  line L41 (-45.4221, 28.5) -> (-45.5636, 28.5) projected
  line L42 (-45.5636, 28.5) -> (-45.5636, 28.5) projected
  line L43 (-45.5636, 28.5) -> (-45.4221, 28.5) projected
  line L44 (-45.4221, 28.5) -> (-45.4221, 28.5) projected
  line L45 (-43.7886, 31.1091) -> (-41.6673, 28.9878) projected
  line L46 (-38.8388, 21.9167) -> (-36.7175, 19.7954) projected
  line L47 (-36.7175, 24.038) -> (-34.5962, 21.9167) projected
  line L48 (-25.3157, 11.1519) -> (-22.7176, 9.6519) projected
  line L49 (-23.8157, 13.75) -> (-21.2176, 12.25) projected
  line L50 (-11.1962, 3) -> (-12.8705, 3.9667) projected
  line L51 (-12.8705, 3.9667) -> (-12.8705, 3.9667) projected
  line L52 (-12.8705, 3.9667) -> (-11.1962, 3) projected
  line L53 (-11.1962, 3) -> (-11.3962, 3) projected
  line L54 (-11.3962, 3) -> (-11.3962, 3) projected
  line L55 (-11.3962, 3) -> (-11.1962, 3) projected
  line L56 (-11.6913, 6.75) -> (-9.0933, 5.25) projected
  line L57 (-236.5, 6) -> (-229.5, 6)
  line L58 (-229.5, 6) -> (-229.5, 3)
  line L59 (-229.5, 3) -> (-236.5, 3)
  line L60 (-236.5, 3) -> (-236.5, 6)
  line L61 (-163.5, 6) -> (-156.5, 6)
  line L62 (-156.5, 6) -> (-156.5, 3)
  line L63 (-156.5, 3) -> (-163.5, 3)
  line L64 (-163.5, 3) -> (-163.5, 6)
  line L65 (-90.5, 3) -> (-90.5, 6)
  line L66 (-83.5, 6) -> (-83.5, 3)
  line L67 (-83.5, 3) -> (-90.5, 3)
  line L68 (-90.5, 6) -> (-83.5, 6)
  line L69 (-292.9308, 12.1643) -> (-298.993, 8.6643)
  line L70 (-297.2609, 9.6643) -> (-294.6629, 11.1643) projected
  line L71 (-298.993, 8.6643) -> (-297.493, 6.0662)
  line L72 (-297.493, 6.0662) -> (-291.4308, 9.5662)
  line L73 (-291.4308, 9.5662) -> (-292.9308, 12.1643)
  line L74 (-27.0477, 12.1519) -> (-20.9856, 8.6519)
  line L75 (-20.9856, 8.6519) -> (-22.4856, 6.0538)
  line L76 (-22.4856, 6.0538) -> (-28.5477, 9.5538)
  line L77 (-28.5477, 9.5538) -> (-27.0477, 12.1519)
  line L78 (-31.842, 14.9199) -> (-11.1962, 3) projected
  line L79 (-31.842, 14.9199) -> (-11.1962, 3) projected
  line L80 (-270, 57) -> (-267, 57) projected
  line L81 (-267, 57) -> (-264, 57)
  line L82 (-242, 57) -> (-270, 57) projected
  line L83 (-264, 57) -> (-264, 75.2541)
  line L84 (-267, 76.0722) -> (-206.5975, 59.5988) projected
  line L85 (-267, 76.0722) -> (-267, 57)
  line L86 (-267, 57) -> (-267, 76.0722) projected
  line L87 (-267, 76.0722) -> (-263.8416, 75.2541)
  line L88 (-53, 57) -> (-56, 57)
  line L89 (-53, 57) -> (-78, 57) projected
  line L90 (-56, 57) -> (-56, 75.2541)
  line L91 (-113.4025, 59.5988) -> (-53, 76.0722) projected
  line L92 (-56, 75.2541) -> (-53, 76.0722)
  line L93 (-53, 76.0722) -> (-53, 57) projected
  line L94 (-53, 76.0722) -> (-53, 57)
  line L95 (-214.4731, 3) -> (-308.8038, 3) projected
  line L96 (-308.8038, 3) -> (-288.158, 14.9199) projected
  line L97 (-302.4992, 3) -> (-302.4992, 6.64)
  line L98 (-302.4992, 3) -> (-298.8592, 3) construction
  line L99 (-302.4992, 6.64) -> (-308.8038, 3)
  line L100 (-214.4731, 3) -> (-308.8038, 3) projected
  line L101 (-308.8038, 3) -> (-302.4992, 3)
  line L102 (-17.5008, 3) -> (-17.5008, 6.64)
  line L103 (-17.5008, 3) -> (-13.8608, 3) construction
  line L104 (-11.1962, 3) -> (-107.5, 3) projected
  line L105 (-31.842, 14.9199) -> (-11.1962, 3) projected
  line L106 (-17.5008, 6.64) -> (-11.1962, 3)
  line L107 (-11.1962, 3) -> (-17.5008, 3)
  line L108 (-11.1962, 3) -> (-107.5, 3) projected
  point P0 (0, 0)
  dimension "d252" = 7
  dimension "d253" = 3
  dimension "d256" = 7
  dimension "d257" = 3
  dimension "d258" = 7
  dimension "d259" = 3
  dimension "d266" = 7
  dimension "d267" = 3
  dimension "d268" = 7
  dimension "d269" = 7
  dimension "d270" = 3
  dimension "d271" = 7
  dimension "d302" = 3.64
  dimension "d303" = 90
  dimension "d304" = 3.64
  dimension "d305" = 90
  constraints: 72 end point, 10 perpendicular, 7 horizontal, 7 parallel, 6 collinear, 5 point on line, 3 vertical, 6 other
  measures "d252" distance of L58.end L59.end
  measures "d253" distance of L57.end L58.end
  measures "d256" distance of L62.end L64.start
  measures "d257" distance of L62.start L62.end
  measures "d258" distance of L66.end L67.end
  measures "d259" distance of L66.start L66.end
  measures "d266" distance of L69.start L69.end
  measures "d267" distance of L69.end L71.end
  measures "d268" distance of L71.end L72.end
  measures "d269" distance of L74.start L74.end
  measures "d270" distance of L74.end L75.end
  measures "d271" distance of L75.end L76.end
  measures "d302" distance of L97.start L97.end
  measures "d303" angle of L98 L97
  measures "d304" distance of L102.start L102.end
  measures "d305" angle of L103 L102
extrude "돌출27" cut sketch "스케치11" against normal blind 6.1 contours A0 L6 L5 | L5 L6 A0 | A4 L9 L10 | L10 L9 A4 | A1 L7 L6 | L6 L7 A1 | A3 L8 L9 | L9 L8 A3 | A2 L8 L7 | L7 L8 A2
extrude "돌출36" add sketch "스케치25" against normal blind 7.3
extrude "돌출29" cut sketch "스케치15" against normal blind 6.1 contours A1 | A6 | A8 | A9
extrude "돌출31" cut sketch "스케치18" against normal blind 6.1 contours A2 | A5 | A8 | A9
sketch "스케치26" plane through (8, 57, -270) normal (0, 0, -1) x (-1, 0, 0)
  circle A0 centre (-36, 17) radius 1.5 projected
  circle A1 centre (4, 17) radius 1.5 projected
  circle A2 centre (223.8, 17) radius 1.5 projected
  circle A3 centre (263.8, 17) radius 1.5 projected
  circle A4 centre (263.8, 7) radius 1.5 projected
  circle A5 centre (223.8, 7) radius 1.5 projected
  circle A6 centre (4, 7) radius 1.5 projected
  circle A7 centre (-36, 7) radius 1.5 projected
  line L0 (153.9, -14) -> (73.9, -14) projected
  line L1 (73.9, -14) -> (73.9, 0) projected
  line L2 (73.9, 0) -> (153.9, 0) projected
  line L3 (153.9, 0) -> (153.9, -14) projected
  line L4 (38.9, 0) -> (38.9, -14) projected
  line L5 (38.9, -14) -> (-31.1, -14) projected
  line L6 (-31.1, -14) -> (-31.1, 0) projected
  line L7 (-31.1, 0) -> (38.9, 0) projected
  line L8 (258.9, -14) -> (188.9, -14) projected
  line L9 (188.9, -14) -> (188.9, 0) projected
  line L10 (188.9, 0) -> (258.9, 0) projected
  line L11 (258.9, 0) -> (258.9, -14) projected
  line L12 (268.9, 23) -> (268.9, -17) projected
  line L13 (-41.1, 23) -> (268.9, 23) projected
  line L14 (-41.1, -17) -> (-41.1, 23) projected
  line L15 (268.9, -17) -> (-41.1, -17) projected
  circle A8 centre (4, 17) radius 1.25
  circle A9 centre (4, 7) radius 1.25
  point P0 (8, -57)
  dimension "d294" = 2.5
  dimension "d295" = 2.5
  constraints: 2 centre point, 2 coincident
  measures "d294" diameter of A8
  measures "d295" diameter of A9
extrude "돌출34" cut sketch "스케치26" against normal blind 6.1 contours A1 | A6 | A8 | A9
sketch "스케치27" plane through (0, 57, -50) normal (0, 0, 1) x (1, 0, 0)
  circle A0 centre (-255.8, 17) radius 1.5 projected
  circle A1 centre (-215.8, 17) radius 1.5 projected
  circle A2 centre (4, 17) radius 1.5 projected
  circle A3 centre (44, 17) radius 1.5 projected
  circle A4 centre (44, 7) radius 1.5 projected
  circle A5 centre (4, 7) radius 1.5 projected
  circle A6 centre (-215.8, 7) radius 1.5 projected
  circle A7 centre (-255.8, 7) radius 1.5 projected
  line L0 (-65.9, -14) -> (-145.9, -14) projected
  line L1 (-145.9, -14) -> (-145.9, 0) projected
  line L2 (-145.9, 0) -> (-65.9, 0) projected
  line L3 (-65.9, 0) -> (-65.9, -14) projected
  line L4 (-180.9, 0) -> (-180.9, -14) projected
  line L5 (-180.9, -14) -> (-250.9, -14) projected
  line L6 (-250.9, -14) -> (-250.9, 0) projected
  line L7 (-250.9, 0) -> (-180.9, 0) projected
  line L8 (39.1, -14) -> (-30.9, -14) projected
  line L9 (-30.9, -14) -> (-30.9, 0) projected
  line L10 (-30.9, 0) -> (39.1, 0) projected
  line L11 (39.1, 0) -> (39.1, -14) projected
  line L12 (49.1, 23) -> (49.1, -17) projected
  line L13 (-260.9, 23) -> (49.1, 23) projected
  line L14 (-260.9, -17) -> (-260.9, 23) projected
  line L15 (49.1, -17) -> (-260.9, -17) projected
  circle A8 centre (4, 17) radius 1.25
  circle A9 centre (4, 7) radius 1.25
  point P0 (0, -57)
  dimension "d298" = 2.5
  dimension "d299" = 2.5
  constraints: 2 centre point, 2 coincident
  measures "d298" diameter of A8
  measures "d299" diameter of A9
extrude "돌출35" cut sketch "스케치27" against normal blind 6.1 contours A2 | A5 | A8 | A9
sketch "스케치28" plane through (0, 0, 0) normal (0, 0.8660254, 0.5) x (1, 0, 0)
  circle A0 centre (-63, 15.5247) radius 1.5 projected
  circle A1 centre (-148.8, 25.5247) radius 1.5 projected
  circle A2 centre (-148.8, 15.5247) radius 1.5 projected
  circle A3 centre (-63, 25.5247) radius 1.5 projected
  circle A4 centre (44, 25.5247) radius 1.5 projected
  circle A5 centre (4, 15.5247) radius 1.5 projected
  circle A6 centre (-215.8, 25.5247) radius 1.5 projected
  circle A7 centre (-255.8, 25.5247) radius 1.5 projected
  circle A8 centre (-255.8, 15.5247) radius 1.5 projected
  circle A9 centre (-215.8, 15.5247) radius 1.5 projected
  circle A10 centre (4, 25.5247) radius 1.5 projected
  circle A11 centre (44, 15.5247) radius 1.5 projected
  line L0 (-97.9, 33.5247) -> (-97.9, 26.5247) projected
  arc A12 (-99.9, 24.5247) -> (-97.9, 26.5247) centre (-99.9, 26.5247) ccw projected
  line L1 (-99.9, 24.5247) -> (-111.9, 24.5247) projected
  arc A13 (-113.9, 26.5247) -> (-111.9, 24.5247) centre (-111.9, 26.5247) ccw projected
  line L2 (-113.9, 26.5247) -> (-113.9, 33.5247) projected
  line L3 (-260.9, 33.5247) -> (-113.9, 33.5247) projected
  line L4 (-260.9, -0.4753) -> (-260.9, 33.5247) projected
  line L5 (49.1, -0.4753) -> (-260.9, -0.4753) projected
  line L6 (49.1, 33.5247) -> (49.1, -0.4753) projected
  line L7 (-97.9, 33.5247) -> (49.1, 33.5247) projected
  circle A14 centre (4, 25.5247) radius 1.25
  circle A15 centre (4, 15.5247) radius 1.25
  point P0 (0, 0)
  dimension "d308" = 2.5
  dimension "d309" = 2.5
  constraints: 2 centre point, 2 coincident
  measures "d308" diameter of A14
  measures "d309" diameter of A15
extrude "돌출37" cut sketch "스케치28" against normal blind 6.1 contours A14 | A15
sketch "스케치29" plane through (0, 17.3205, -290) normal (0, 0.8660254, -0.5) x (1, 0, 0)
  circle A0 centre (-148.8, 19.1163) radius 1.5 projected
  circle A1 centre (-63, 9.1163) radius 1.5 projected
  circle A2 centre (-63, 19.1163) radius 1.5 projected
  circle A3 centre (-148.8, 9.1163) radius 1.5 projected
  circle A4 centre (-255.8, 9.1163) radius 1.5 projected
  circle A5 centre (-215.8, 19.1163) radius 1.5 projected
  circle A6 centre (4, 9.1163) radius 1.5 projected
  circle A7 centre (44, 9.1163) radius 1.5 projected
  circle A8 centre (44, 19.1163) radius 1.5 projected
  circle A9 centre (4, 19.1163) radius 1.5 projected
  circle A10 centre (-215.8, 9.1163) radius 1.5 projected
  circle A11 centre (-255.8, 19.1163) radius 1.5 projected
  line L0 (-113.9, 1.1163) -> (-113.9, 8.1163) projected
  arc A12 (-111.9, 10.1163) -> (-113.9, 8.1163) centre (-111.9, 8.1163) ccw projected
  line L1 (-111.9, 10.1163) -> (-99.9, 10.1163) projected
  arc A13 (-97.9, 8.1163) -> (-99.9, 10.1163) centre (-99.9, 8.1163) ccw projected
  line L2 (-97.9, 8.1163) -> (-97.9, 1.1163) projected
  line L3 (49.1, 1.1163) -> (-97.9, 1.1163) projected
  line L4 (49.1, 35.1163) -> (49.1, 1.1163) projected
  line L5 (-260.9, 35.1163) -> (49.1, 35.1163) projected
  line L6 (-260.9, 1.1163) -> (-260.9, 35.1163) projected
  line L7 (-113.9, 1.1163) -> (-260.9, 1.1163) projected
  circle A14 centre (4, 9.1163) radius 1.25
  circle A15 centre (4, 19.1163) radius 1.25
  point P0 (0, -242.4871)
  dimension "d312" = 2.5
  dimension "d313" = 2.5
  constraints: 2 centre point, 2 coincident
  measures "d312" diameter of A14
  measures "d313" diameter of A15
extrude "돌출38" cut sketch "스케치29" against normal blind 6.1 contours A14 | A15
sketch "스케치30" plane through (8, 0, 0) normal (1, 0, 0) x (0, 0, -1)
  circle A0 centre (211, 27) radius 12.6 projected
  circle A1 centre (211, 9.4) radius 2.1 projected
  circle A2 centre (211, 44.6) radius 2.1 projected
  circle A3 centre (193.4, 27) radius 2.1 projected
  circle A4 centre (228.6, 27) radius 2.1 projected
  arc A5 (39, 20.3205) -> (37, 18.3205) centre (39, 18.3205) ccw projected
  line L0 (39, 20.3205) -> (48, 20.3205) projected
  arc A6 (50, 18.3205) -> (48, 20.3205) centre (48, 18.3205) ccw projected
  line L1 (50, 18.3205) -> (50, 14.3205) projected
  arc A7 (48, 12.3205) -> (50, 14.3205) centre (48, 14.3205) ccw projected
  line L2 (48, 12.3205) -> (39, 12.3205) projected
  arc A8 (37, 14.3205) -> (39, 12.3205) centre (39, 14.3205) ccw projected
  line L3 (37, 14.3205) -> (37, 18.3205) projected
  arc A9 (272, 20.3205) -> (270, 18.3205) centre (272, 18.3205) ccw projected
  line L4 (272, 20.3205) -> (281, 20.3205) projected
  arc A10 (283, 18.3205) -> (281, 20.3205) centre (281, 18.3205) ccw projected
  line L5 (283, 18.3205) -> (283, 14.3205) projected
  arc A11 (281, 12.3205) -> (283, 14.3205) centre (281, 14.3205) ccw projected
  line L6 (281, 12.3205) -> (272, 12.3205) projected
  arc A12 (270, 14.3205) -> (272, 12.3205) centre (272, 14.3205) ccw projected
  line L7 (270, 14.3205) -> (270, 18.3205) projected
  circle A13 centre (109, 27) radius 7.55 projected
  arc A14 (166, 38) -> (164, 40) centre (164, 38) ccw projected
  line L8 (166, 38) -> (166, 20) projected
  arc A15 (164, 18) -> (166, 20) centre (164, 20) ccw projected
  line L9 (164, 18) -> (156, 18) projected
  arc A16 (154, 20) -> (156, 18) centre (156, 20) ccw projected
  line L10 (154, 20) -> (154, 38) projected
  arc A17 (156, 40) -> (154, 38) centre (156, 38) ccw projected
  line L11 (156, 40) -> (164, 40) projected
  circle A18 centre (160, 14.5) radius 1.5 projected
  circle A19 centre (160, 43.5) radius 1.5 projected
  line L12 (270, 80) -> (160, 50) projected
  line L13 (160, 50) -> (50, 80) projected
  line L14 (50, 80) -> (50, 57) projected
  line L15 (50, 57) -> (78, 57) projected
  arc A20 (80, 55) -> (78, 57) centre (78, 55) ccw projected
  line L16 (80, 55) -> (80, 45) projected
  arc A21 (78, 43) -> (80, 45) centre (78, 45) ccw projected
  line L17 (78, 43) -> (50, 43) projected
  line L18 (50, 43) -> (50, 37.3205) projected
  line L19 (50, 37.3205) -> (30, 17.3205) projected
  line L20 (30, 17.3205) -> (0, 0) projected
  line L21 (0, 0) -> (320, 0) projected
  line L22 (320, 0) -> (290, 17.3205) projected
  line L23 (290, 17.3205) -> (270, 37.3205) projected
  line L24 (270, 37.3205) -> (270, 43) projected
  line L25 (270, 43) -> (242, 43) projected
  arc A22 (240, 45) -> (242, 43) centre (242, 45) ccw projected
  line L26 (240, 45) -> (240, 55) projected
  arc A23 (242, 57) -> (240, 55) centre (242, 55) ccw projected
  line L27 (242, 57) -> (270, 57) projected
  line L28 (270, 57) -> (270, 80) projected
  line L29 (133, 0) -> (133, 43.5)
  line L30 (133, 0) -> (176.5, 0) construction
  circle A24 centre (133, 43.5) radius 1.5
  circle A25 centre (133, 37.5) radius 1.5
  circle A26 centre (133, 31.5) radius 1.5
  dimension "d316" = 43.5
  dimension "d317" = 90
  dimension "d318" = 21
  dimension "d319" = 3
  dimension "d320" = 3
  dimension "d321" = 3
  dimension "d322" = 6
  dimension "d323" = 6
  constraints: 4 end point, 3 centre point, 3 point on line, 1 coincident, 1 horizontal, 1 perpendicular, 1 vertical
  measures "d316" distance of L29.start L29.end
  measures "d317" angle of L30 L29
  measures "d318" distance between parallel lines of L10 L29
  measures "d319" diameter of A24
  measures "d320" diameter of A25
  measures "d321" diameter of A26
  measures "d322" distance of A25.centre L29.end
  measures "d323" distance of A26.centre A25.centre
extrude "돌출39" cut sketch "스케치30" against normal blind 2 contours A26 L29 | L29 A26 | A25 L29 | L29 A25 | A24